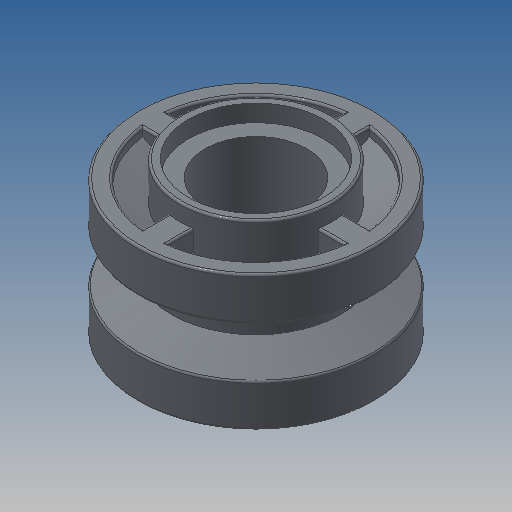
# Autodesk Inventor part: 42610-LtBluishGray
Saved by Autodesk Inventor 2022.2 (Build 262287000, 287)
## iProperties
Created: 2014-08-18
Part Number: 42610-LtBluishGray
Material: ABS Plastic
Document SubType Name: Modeling
Designer: D. Kohfeld
Density: 1.06 g/cm^3
Appearance: LtBluishGray
Mass: 0.438059 g
Surface Area: 6.61207 cm^2
Volume: 0.413263 cm^3
Author: D. Kohfeld
Autodesk Inventor part; units mm, degrees
ref_plane "YZ Plane" through (0, 0, 0) normal (1, 0, 0) x (0, 1, 0)
ref_plane "XZ Plane" through (0, 0, 0) normal (0, 1, 0) x (-1, 0, 0)
ref_plane "XY Plane" through (0, 0, 0) normal (0, 0, 1) x (1, 0, 0)
sketch "Sketch2" plane through (0, 0, 0) normal (1, 0, 0) x (0, 1, 0)
  line L0 (-1.2, -5.6) -> (-0.4, -4)
  line L1 (-0.4, -4) -> (0.4, -4)
  line L2 (0.4, -4) -> (1.2, -5.6)
  line L3 (1.2, -5.6) -> (3.2, -5.6)
  line L4 (3.2, -5.6) -> (3.2, -4.8)
  line L5 (3.2, -4.8) -> (2.8, -4.8)
  line L6 (2.8, -4.8) -> (2.2, -3.6)
  line L7 (2.2, -3.6) -> (4, -3.6)
  line L8 (4, -3.6) -> (4, -3.2)
  line L9 (4, -3.2) -> (3.2, -3.2)
  line L10 (3.2, -3.2) -> (3.2, -2.4)
  line L11 (3.2, -2.4) -> (-3.2, -2.4)
  line L12 (-3.2, -2.4) -> (-3.2, -3.2)
  line L13 (-3.2, -3.2) -> (-4, -3.2)
  line L14 (-4, -3.2) -> (-4, -3.6)
  line L15 (-4, -3.6) -> (-2.2, -3.6)
  line L16 (-2.2, -3.6) -> (-2.8, -4.8)
  line L17 (-2.8, -4.8) -> (-3.2, -4.8)
  line L18 (-3.2, -4.8) -> (-3.2, -5.6)
  line L19 (-3.2, -5.6) -> (-1.2, -5.6)
  line L20 (-5.6, 0) -> (5.6, 0) projected
  point P0 (0, 0)
  point P1 (0, -2.4)
  dimension "d0" = 4.8
  dimension "d1" = 6.4
  dimension "d2" = 0.8
  dimension "d3" = 8
  dimension "d4" = 7.2
  dimension "d5" = 11.2
  dimension "d6" = 9.6
  dimension "d7" = 6.4
  dimension "d8" = 0.8
  dimension "d9" = 8
  dimension "d10" = 0.4
  dimension "d11" = 2.4
  constraints: 40 end point, 13 parallel, 8 equal length, 3 perpendicular, 1 collinear, 1 horizontal, 1 horizontal alignment, 1 midpoint, 1 vertical alignment
  measures "d0" diameter of L11 L20
  measures "d1" diameter of L9 L20
  measures "d2" distance between parallel lines of L10 L8
  measures "d3" distance between parallel lines of L14 L8
  measures "d4" diameter of L7 L20
  measures "d5" diameter of L19 L20
  measures "d6" diameter of L17 L20
  measures "d7" distance between parallel lines of L4 L18
  measures "d8" distance of L0.end L1.end
  measures "d9" diameter of L1 L20
  measures "d10" distance from line of L5.end L4
  measures "d11" distance of L2.end L0.start
revolve "Revolution1" add sketch "Sketch2" angle 360 about axis through (0, -10, 0) along (0, 1, 0)
sketch "Sketch3" plane through (0, 3.2, 0) normal (0, 1, 0) x (1, 0, 0)
  circle A0 centre (0, 0) radius 4.8 projected
  circle A1 centre (0, 0) radius 3.6 projected
  line L0 (-0.6, 4.7624) -> (-0.6, 3.5496)
  line L1 (0.6, 3.5496) -> (0.6, 4.7624)
  line L2 (-3.5496, 0.6) -> (-4.7624, 0.6)
  line L3 (-4.7624, -0.6) -> (-3.5496, -0.6)
  line L4 (-0.6, -3.5496) -> (-0.6, -4.7624)
  line L5 (0.6, -3.5496) -> (0.6, -4.7624)
  line L6 (3.5496, -0.6) -> (4.7624, -0.6)
  line L7 (3.5496, 0.6) -> (4.7624, 0.6)
  dimension "d14" = 1.2
  constraints: 16 end point, 7 equal length, 3 parallel, 3 perpendicular, 2 vertical, 18 other
  measures "d14" distance between parallel lines of L0 L1
extrude "Extrusion1" add sketch "Sketch3" against normal up to next contours A0 L6 A1 L7 | L1 A1 L0 A0 | A0 L4 A1 L5 | L2 A1 L3 A0
mirror "Mirror1" about plane through (0, 0, 0) normal (0, 1, 0) of "Extrusion1"
fillet "Fillet1" radius 0.1 30 edges at (0, 4, 3.6) (-0.6, 3.2, 4.156) (3.3941, 3.2, 3.3941) (0.6, 3.2, 4.156) (-3.3941, 3.2, 3.3941) (-4.156, 3.2, 0.6) (-4.156, 3.2, -0.6) (-3.3941, 3.2, -3.3941) (-0.6, 3.2, -4.156) (0.6, 3.2, -4.156) (3.3941, 3.2, -3.3941) (4.156, 3.2, -0.6) (4.156, 3.2, 0.6) (0, 1.2, 5.6) (0, 3.2, 5.6) (0, -1.2, 5.6) (0, -3.2, 5.6) (4.156, -3.2, 0.6) (3.3941, -3.2, 3.3941) (0.6, -3.2, 4.156) (-0.6, -3.2, 4.156) (-3.3941, -3.2, 3.3941) (-4.156, -3.2, 0.6) (-4.156, -3.2, -0.6) (-3.3941, -3.2, -3.3941) (-0.6, -3.2, -4.156) (0.6, -3.2, -4.156) (3.3941, -3.2, -3.3941) (4.156, -3.2, -0.6) (0, -4, 3.6)
equation "\"d0\" = tpd"
equation "\"d1\" = tsd"
equation "\"d2\" = tsl"
equation "\"d3\" = lu"
equation "\"d4\" = tlad"
equation "\"d9\" = lu"
equation "\"d17\" = lf"
equation "\"tpd\" = 4.8"
equation "\"tsd\" = 6.4"
equation "\"tsl\" = 0.8"
equation "\"lu\" = 8"
equation "\"tlad\" = 7.2"
equation "\"lf\" = 0.1"
body "Solid1"
